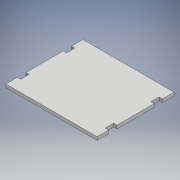
# Autodesk Inventor part: TAPA_CAJA
Saved by Autodesk Inventor 2018 (Build 220112000, 112)
## iProperties
Created: 2018-03-07
Part Number: TAPA_CAJA
Material: Generic
Document SubType Name: Modeling
Designer: isai
Density: 1 g/cm^3
Appearance: Default
Author: isai
Autodesk Inventor part; units mm, degrees
ref_plane "YZ Plane" through (0, 0, 0) normal (1, 0, 0) x (0, 1, 0)
ref_plane "XZ Plane" through (0, 0, 0) normal (0, 1, 0) x (-1, 0, 0)
ref_plane "XY Plane" through (0, 0, 0) normal (0, 0, 1) x (1, 0, 0)
sketch "Sketch1" plane through (0, 0, 0) normal (0, 0, 1) x (1, 0, 0)
  line L0 (0, -24) -> (0, -14)
  line L1 (4, -14) -> (4, -24)
  line L2 (0, -79) -> (0, -69)
  line L3 (4, -69) -> (4, -79)
  line L4 (0, -69) -> (4, -69)
  line L5 (0, -79) -> (4, -79)
  line L6 (106, -79) -> (106, -69)
  line L7 (110, -69) -> (110, -79)
  line L8 (110, -14) -> (106, -14)
  line L9 (110, -24) -> (106, -24)
  line L10 (106, -24) -> (106, -14)
  line L11 (110, -14) -> (110, -24)
  line L12 (0, 0) -> (110, 0)
  line L13 (110, 0) -> (110, -93)
  line L14 (110, -93) -> (0, -93)
  line L15 (0, -93) -> (0, 0)
  line L16 (4, -14) -> (0, -14)
  line L17 (0, -14) -> (0, -24)
  line L18 (0, -24) -> (4, -24)
  line L19 (4, -24) -> (4, -14)
  line L20 (106, -69) -> (110, -69)
  line L21 (110, -69) -> (110, -79)
  line L22 (110, -79) -> (106, -79)
  line L23 (106, -79) -> (106, -69)
  constraints: 48 end point, 6 parallel, 3 horizontal, 3 perpendicular
extrude "Extrusion1" add sketch "Sketch1" along normal blind 4 contours L18 L1 L16 L15 L12 L13 L8 L10 L9 L20 L6 L22 L14 L5 L3 L4
body "Solid1"
